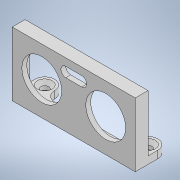
# Autodesk Inventor part: Крепление ультрасоника
Saved by Autodesk Inventor 2020 (Build 240168000, 168)
## iProperties
Created: 2021-05-10
Part Number: Крепление ультрасоника
Material: Типовые
Document SubType Name: Modeling
Designer: Антон
Density: 1 g/cm^3
Appearance: По умолчанию
Author: Антон
Autodesk Inventor part; units mm, degrees
sketch "Эскиз1" plane through (0, 0, 0) normal (0, 0, 1) x (1, 0, 0)
  line L0 (0, 0) -> (50, 0)
  line L1 (50, 0) -> (50, 25)
  line L2 (50, 25) -> (0, 25)
  line L3 (0, 25) -> (0, 0)
  dimension "d0" = 50
  dimension "d1" = 25
  constraints: 8 end point, 2 parallel, 1 horizontal, 1 perpendicular
  measures "d0" distance of L2.end L1.end
  measures "d1" distance of L1.end L0.end
extrude "Выдавливание1" add sketch "Эскиз1" along normal blind 5.2
shell "Оболочка1" thickness 2 removed faces 1 at (16.6667, 16.6667, 0)
sketch "Эскиз2" plane through (0, 0, 5.2) normal (0, 0, 1) x (1, 0, 0)
  line L0 (50, 25) -> (0, 25) projected
  line L1 (25, 25) -> (25, 0)
  line L2 (0, 0) -> (50, 0) projected
  line L3 (25, 12.5) -> (12, 12.5)
  line L4 (0, 25) -> (0, 0) projected
  circle A0 centre (12, 12.5) radius 8.1
  circle A1 centre (38, 12.5) radius 8.1
  line L5 (25, 25) -> (25, 20)
  line L6 (21.75, 20) -> (28.25, 20) construction
  line L7 (21.75, 18) -> (28.25, 18)
  line L8 (28.25, 22) -> (21.75, 22)
  arc A2 (21.75, 22) -> (21.75, 18) centre (21.75, 20) ccw
  arc A3 (28.25, 18) -> (28.25, 22) centre (28.25, 20) ccw
  point P0 (25, 18)
  point P1 (25, 22)
  dimension "d5" = 13
  dimension "d6" = 16.2
  dimension "d9" = 5
  dimension "d10" = 3.25
  dimension "d11" = 4
  constraints: 14 end point, 4 centre point, 4 midpoint, 4 point on circle, 4 tangent, 1 coincident, 1 horizontal, 1 parallel, 1 perpendicular, 1 point on line, 1 symmetric about line, 1 other
  measures "d5" distance of L3.start L3.end
  measures "d6" diameter of A0
  measures "d9" distance of L1.start L5.end
  measures "d10" distance of L5.end L6.end
  measures "d11" diameter of A3
extrude "Выдавливание2" cut sketch "Эскиз2" against normal through all contours L8 A3 L7 L1 | L1 L7 A2 L8 | A0 | A1
sketch "Эскиз5" plane through (48, 23, 3.2) normal (0, 0, -1) x (-1, 0, 0)
  line L0 (0, 0) -> (1.05, 0)
  line L1 (0, 0) -> (46, 0) projected
  line L2 (1.05, 0) -> (1.05, -1.05)
  circle A0 centre (1.05, -1.05) radius 1.05
  line L3 (2.1, -2.1) -> (0, -2.1)
  line L4 (0, -2.1) -> (0, 0)
  line L5 (0, 0) -> (2.1, 0)
  line L6 (2.1, 0) -> (2.1, -2.1)
  line L7 (2.1, -2.1) -> (0, 0) construction
  line L8 (0, -2.1) -> (2.1, 0) construction
  point P0 (48, -23)
  point P1 (1.05, -2.1)
  point P2 (2.1, -1.05)
  dimension "d17" = 1.05
  dimension "d18" = 1.05
  constraints: 16 end point, 2 midpoint, 2 parallel, 1 coincident, 1 horizontal, 1 perpendicular, 1 point on line, 1 vertical, 3 other
  measures "d17" distance of L0.start L0.end
  measures "d18" distance of L0.end L2.end
extrude "Выдавливание4" add sketch "Эскиз5" along normal blind 1 contours L0 A0 L4 | L1 L6 A0 | A0 | A0 L3 L4
ref_plane "РабПлоскость1" through (25, 2, 0) normal (1, 0, 0) x (0, 0, -1)
ref_plane "РабПлоскость2" through (2, 12.5, 0) normal (0, -1, 0) x (1, 0, 0)
mirror "Зеркальное отражение1" about plane through (2, 12.5, 0) normal (0, -1, 0) of "Выдавливание4"
mirror "Зеркальное отражение2" about plane through (25, 2, 0) normal (1, 0, 0) of "Выдавливание4", "Зеркальное отражение1"
sketch "Эскиз10" plane through (0, 0, 0) normal (0, -1, 0) x (1, 0, 0)
  line L0 (0, 0) -> (50, 0) projected
  line L1 (50, 0) -> (42, 0)
  line L2 (42, 0) -> (42, -8)
  line L3 (42, -8) -> (50, -8)
  line L4 (50, -8) -> (50, 0)
  dimension "d39" = 8
  dimension "d40" = 8
  constraints: 8 end point, 2 parallel, 1 horizontal, 1 perpendicular
  measures "d39" distance of L3.end L2.end
  measures "d40" distance of L2.end L1.end
extrude "Выдавливание8" add sketch "Эскиз10" against normal up to surface (2 mm away)
sketch "Эскиз11" plane through (48, 2, 0) normal (0, 1, 0) x (1, 0, 0)
  line L0 (-6, 0) -> (-6, 8) projected
  line L1 (-6, 4) -> (2, 4)
  line L2 (2, 0) -> (2, 8) projected
  line L3 (-6, 8) -> (-6, 0) projected
  point P0 (-48, 0)
  point P1 (-2, 4)
  constraints: 3 midpoint, 2 end point, 1 perpendicular
hole "Отверстие2" at (46, 2, -4) direction (0, -1, 0) diameter 3.2 end through all countersink diameter 6 countersink angle 90
ref_plane "РабПлоскость3" through (25, 25, 5.2) normal (1, 0, 0) x (0, 0, -1)
mirror "Зеркальное отражение4" about plane through (25, 25, 5.2) normal (1, 0, 0) of "Отверстие2", "Выдавливание8"
fillet "Сопряжение2" radius 4 6 edges at (42, 1, -8) (50, 1, -8) (8, 1, -8) (0, 1, -8) (8, 1, 0) (42, 1, 0)
sketch "Эскиз12" plane through (0, 0, 5.2) normal (0, -1, 0) x (1, 0, 0)
  circle A0 centre (46, -9.2) radius 1.6 projected
  circle A1 centre (4, -9.2) radius 1.6 projected
  arc A2 (0, -9.2) -> (8, -9.2) centre (4, -9.2) ccw projected
  arc A3 (12, -5.2) -> (8, -9.2) centre (12, -9.2) ccw projected
  line L0 (12, -5.2) -> (38, -5.2) projected
  arc A4 (42, -9.2) -> (38, -5.2) centre (38, -9.2) ccw projected
  arc A5 (42, -9.2) -> (50, -9.2) centre (46, -9.2) ccw projected
  line L1 (50, -9.2) -> (50, 0) projected
  line L2 (0, 0) -> (50, 0) projected
  line L3 (0, -9.2) -> (0, 0) projected
  point P0 (0, -5.2)
extrude "Выдавливание9" add sketch "Эскиз12" along normal blind 1
